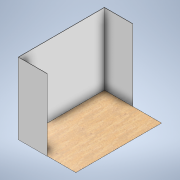
# Autodesk Inventor part: Monter
Saved by Autodesk Inventor 2020 (Build 240168000, 168)
## iProperties
Created: 2020-02-17
Part Number: Monter
Material: Generic
Document SubType Name: Modeling
Designer: Patrik
Density: 1 g/cm^3
Appearance: Monter Vägg
Author: Patrik
Autodesk Inventor part; units mm, degrees
ref_plane "YZ Plane" through (0, 0, 0) normal (1, 0, 0) x (0, 1, 0)
ref_plane "XZ Plane" through (0, 0, 0) normal (0, 1, 0) x (-1, 0, 0)
ref_plane "XY Plane" through (0, 0, 0) normal (0, 0, 1) x (1, 0, 0)
sketch "Sketch1" plane through (0, 0, 0) normal (0, 1, 0) x (-1, 0, 0)
  line L0 (0, 0) -> (2000, 0)
  line L1 (2000, 0) -> (2000, -3000)
  line L2 (2000, -3000) -> (0, -3000)
  line L3 (0, -3000) -> (0, 0)
  dimension "d2" = 2000
  dimension "d3" = 3000
  constraints: 8 end point, 2 parallel, 1 horizontal, 1 perpendicular
  measures "d2" distance of L1.end L2.end
  measures "d3" distance of L0.end L1.end
extrude "Extrusion2" add sketch "Sketch1" along normal blind 1
sketch "Sketch3" plane through (0, 1, 0) normal (0, 1, 0) x (1, 0, 0)
  line L0 (-2000, 0) -> (0, 0) projected
  line L1 (-2000, 0) -> (-1000, 0)
  line L2 (-1000, 0) -> (-1000, -10)
  line L3 (-1000, -10) -> (-2000, -10)
  line L4 (-2000, -10) -> (-2000, 0)
  line L5 (-2000, -10) -> (-2010, -10)
  line L6 (-2010, -10) -> (-2010, 3000)
  line L7 (-2010, 3000) -> (-2000, 3000)
  line L8 (-2000, 3000) -> (-2000, -10)
  line L9 (-2010, 3000) -> (-1010, 3000)
  line L10 (-1010, 3000) -> (-1010, 3010)
  line L11 (-1010, 3010) -> (-2010, 3010)
  line L12 (-2010, 3010) -> (-2010, 3000)
  dimension "d6" = 10
  dimension "d7" = 10
  dimension "d8" = 1000
  dimension "d9" = 1000
  dimension "d10" = 10
  constraints: 24 end point, 6 parallel, 3 horizontal, 3 perpendicular
  measures "d6" distance of L1.end L2.end
  measures "d7" distance of L6.end L7.end
  measures "d8" distance of L2.end L3.end
  measures "d9" distance of L11.end L10.end
  measures "d10" distance of L10.end L9.end
extrude "Extrusion3" add sketch "Sketch3" along normal blind 2500
body "Solid2"
